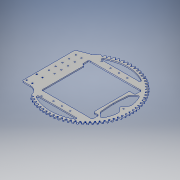
# Autodesk Inventor part: Bearing Plate
Saved by Autodesk Inventor 2019.4 (Build 234330000, 330)
## iProperties
Created: 2020-01-22
Part Number: Bearing Plate
Material: Aluminum 6061
Document SubType Name: Modeling
Designer: admin
Density: 2.7 g/cm^3
Appearance: Aluminum - Flat
Mass: 847.199 g
Surface Area: 1421.78 cm^2
Volume: 313.778 cm^3
Author: admin
Autodesk Inventor part; units mm, degrees
(part 1 of 6)
ref_plane "YZ Plane" through (0, 0, 0) normal (1, 0, 0) x (0, 1, 0)
ref_plane "XZ Plane" through (0, 0, 0) normal (0, 1, 0) x (-1, 0, 0)
ref_plane "XY Plane" through (0, 0, 0) normal (0, 0, 1) x (1, 0, 0)
sketch "Sketch1" plane through (0, 0, 0) normal (0, 1, 0) x (-1, 0, 0)
  arc A0 (63.1453, -163.2105) -> (129.2323, 118) centre (0, 0) ccw construction
  circle A1 centre (0, 0) radius 101.6 construction
  line L0 (-100.2, 110.3) -> (100.2, 110.3)
  line L1 (100.2, 110.3) -> (100.2, -110.3)
  line L2 (100.2, -110.3) -> (-100.2, -110.3)
  line L3 (-100.2, -110.3) -> (-100.2, 110.3)
  line L4 (-100.2, 110.3) -> (100.2, -110.3) construction
  line L5 (100.2, 110.3) -> (-100.2, -110.3) construction
  line L6 (180, 118) -> (180, -118)
  line L7 (180, -118) -> (63.1453, -163.2105)
  line L8 (180, 0) -> (0, 0)
  line L9 (180, 118) -> (129.2323, 118)
  arc A2 (129.2323, 118) -> (63.1453, -163.2105) centre (0, 0) ccw
  dimension "d0" = 350
  dimension "d1" = 203.2
  dimension "d4" = 220.6
  dimension "d5" = 200.4
  dimension "d6" = 180
  dimension "d7" = 118
  constraints: 20 end point, 4 point on circle, 3 centre point, 3 midpoint, 2 coincident, 2 horizontal, 2 parallel, 2 perpendicular, 1 tangent, 1 vertical
  measures "d0" diameter of A0
  measures "d1" diameter of A1
  measures "d4" distance of L2.end L0.start
  measures "d5" distance of L0.start L0.end
  measures "d6" distance from line of point (0, 0) L6
  measures "d7" distance from line of point (0, 0) L9
extrude "Extrusion1" add sketch "Sketch1" along normal blind 5
sketch "Sketch2" plane through (0, 0, 0) normal (0, -1, 0) x (1, 0, 0)
  circle A0 centre (-172.1762, 60.275) radius 2.0193 construction
  circle A1 centre (-172.1762, 105.1064) radius 2.0193 construction
  circle A2 centre (-146.7762, 105.1064) radius 2.0193 construction
  circle A3 centre (-146.7762, 60.275) radius 2.0193 construction
  circle A4 centre (-172.1762, 105.1064) radius 3
  circle A5 centre (-146.7762, 105.1064) radius 3
  circle A6 centre (-146.7762, 60.275) radius 3
  circle A7 centre (-172.1762, 60.275) radius 3
  point P0 (0, 0)
  dimension "d75" = 6
  dimension "d76" = 6
  dimension "d77" = 6
  dimension "d78" = 6
  constraints: 4 centre point, 4 coincident
  measures "d75" diameter of A4
  measures "d76" diameter of A5
  measures "d77" diameter of A6
  measures "d78" diameter of A7
extrude "Extrusion2" cut sketch "Sketch2" against normal through all
chamfer "Chamfer1" distance 3 angle 45 4 edges at (-175.1762, 0, 60.275) (-149.7762, 0, 60.275) (-149.7762, 0, 105.1064) (-175.1762, 0, 105.1064)
sketch "Sketch3" plane through (0, 5, 0) normal (0, 1, 0) x (1, 0, 0)
  line L0 (154.7299, 0) -> (-77.3649, -134) construction
  line L1 (-77.3649, -134) -> (-77.3649, 134) construction
  line L2 (-77.3649, 134) -> (154.7299, 0) construction
  circle A0 centre (-77.3649, 134) radius 2.75
  circle A1 centre (-77.3649, -134) radius 2.75
  circle A2 centre (154.7299, 0) radius 2.75
  point P0 (0, 0)
  point P1 (0, 0)
  dimension "d17" = 268
  dimension "d18" = 5.5
  dimension "d19" = 5.5
  dimension "d20" = 5.5
  constraints: 6 end point, 4 coincident, 3 centre point, 1 vertical, 7 other
  measures "d17" distance of L1.end L0.start
  measures "d18" diameter of A0
  measures "d19" diameter of A1
  measures "d20" diameter of A2
extrude "Extrusion3" cut sketch "Sketch3" against normal through all
sketch "Sketch4" plane through (0, 5, 0) normal (0, 1, 0) x (1, 0, 0)
  circle A0 centre (0, 0) radius 191.0078 construction
  arc A1 (190.8769, -4.9983) -> (190.3537, -14.9812) centre (190.746, -9.9966) ccw
  arc A2 (190.746, -9.9966) -> (201.0078, 0) centre (191.0078, 0) ccw
  arc A3 (199.9066, -21.011) -> (190.746, -9.9966) centre (189.9614, -19.9657) ccw
  line L0 (0, 0) -> (199.9066, -21.011) construction
  arc A4 (189.3088, -24.923) -> (193.6558, -29.9343) centre (188.6561, -29.8802) ccw construction
  line L1 (0, 0) -> (201.0078, 0)
  arc A5 (195.7441, 9.8581) -> (190.8769, 4.9983) centre (190.746, 9.9966) ccw construction
  arc A6 (189.3088, -24.923) -> (190.3537, -14.9812) centre (189.9614, -19.9657) ccw
  arc A7 (190.8769, -4.9983) -> (190.8769, 4.9983) centre (191.0078, 0) ccw
  arc A8 (-129.2323, -118) -> (-63.1453, 163.2105) centre (0, 0) ccw projected
  line L2 (196.0078, 0) -> (175, 0)
  line L3 (194.934, -20.4884) -> (174.0413, -18.2925)
  arc A9 (201.0078, 0) -> (190.746, 9.9966) centre (191.0078, 0) ccw
  arc A10 (190.746, 9.9966) -> (199.9066, 21.011) centre (189.9614, 19.9657) ccw
  arc A11 (199.9066, 21.011) -> (188.6561, 29.8802) centre (189.9614, 19.9657) ccw
  arc A12 (188.6561, 29.8802) -> (196.6152, 41.7919) centre (186.8338, 39.7127) ccw
  arc A13 (196.6152, 41.7919) -> (184.4993, 49.4364) centre (186.8338, 39.7127) ccw
  arc A14 (184.4993, 49.4364) -> (191.1697, 62.1148) centre (181.6592, 59.0246) ccw
  arc A15 (191.1697, 62.1148) -> (178.3211, 68.4511) centre (181.6592, 59.0246) ccw
  arc A16 (178.3211, 68.4511) -> (183.6297, 81.7572) centre (174.4943, 77.6899) ccw
  arc A17 (183.6297, 81.7572) -> (170.1892, 86.7157) centre (174.4943, 77.6899) ccw
  arc A18 (170.1892, 86.7157) -> (174.0778, 100.5039) centre (165.4176, 95.5039) ccw
  arc A19 (174.0778, 100.5039) -> (160.1926, 104.0303) centre (165.4176, 95.5039) ccw
  arc A20 (160.1926, 104.0303) -> (162.6187, 118.1494) centre (154.5285, 112.2715) ccw
  arc A21 (162.6187, 118.1494) -> (148.4409, 120.2051) centre (154.5285, 112.2715) ccw
  arc A22 (148.4409, 120.2051) -> (149.3779, 134.5004) centre (141.9464, 127.8091) ccw
  arc A23 (149.3779, 134.5004) -> (135.0629, 135.0629) centre (141.9464, 127.8091) ccw
  arc A24 (135.0629, 135.0629) -> (134.5004, 149.3779) centre (127.8091, 141.9464) ccw
  arc A25 (134.5004, 149.3779) -> (120.2051, 148.4409) centre (127.8091, 141.9464) ccw
  arc A26 (120.2051, 148.4409) -> (118.1494, 162.6187) centre (112.2715, 154.5285) ccw
  arc A27 (118.1494, 162.6187) -> (104.0303, 160.1926) centre (112.2715, 154.5285) ccw
  arc A28 (104.0303, 160.1926) -> (100.5039, 174.0778) centre (95.5039, 165.4176) ccw
  arc A29 (100.5039, 174.0778) -> (86.7157, 170.1892) centre (95.5039, 165.4176) ccw
  arc A30 (86.7157, 170.1892) -> (81.7572, 183.6297) centre (77.6899, 174.4943) ccw
  arc A31 (81.7572, 183.6297) -> (68.4511, 178.3211) centre (77.6899, 174.4943) ccw
  arc A32 (68.4511, 178.3211) -> (62.1148, 191.1697) centre (59.0246, 181.6592) ccw
  arc A33 (62.1148, 191.1697) -> (49.4364, 184.4993) centre (59.0246, 181.6592) ccw
  arc A34 (49.4364, 184.4993) -> (41.7919, 196.6152) centre (39.7127, 186.8338) ccw
  arc A35 (41.7919, 196.6152) -> (29.8802, 188.6561) centre (39.7127, 186.8338) ccw
  arc A36 (29.8802, 188.6561) -> (21.011, 199.9066) centre (19.9657, 189.9614) ccw
  arc A37 (21.011, 199.9066) -> (9.9966, 190.746) centre (19.9657, 189.9614) ccw
  arc A38 (9.9966, 190.746) -> (0, 201.0078) centre (0, 191.0078) ccw
  arc A39 (0, 201.0078) -> (-9.9966, 190.746) centre (0, 191.0078) ccw
  arc A40 (-9.9966, 190.746) -> (-21.011, 199.9066) centre (-19.9657, 189.9614) ccw
  arc A41 (-21.011, 199.9066) -> (-29.8802, 188.6561) centre (-19.9657, 189.9614) ccw
  arc A42 (-29.8802, 188.6561) -> (-41.7919, 196.6152) centre (-39.7127, 186.8338) ccw
  arc A43 (-41.7919, 196.6152) -> (-49.4364, 184.4993) centre (-39.7127, 186.8338) ccw
  arc A44 (-49.4364, 184.4993) -> (-62.1148, 191.1697) centre (-59.0246, 181.6592) ccw
  arc A45 (-62.1148, 191.1697) -> (-68.4511, 178.3211) centre (-59.0246, 181.6592) ccw
  arc A46 (-68.4511, 178.3211) -> (-81.7572, 183.6297) centre (-77.6899, 174.4943) ccw
  arc A47 (-81.7572, 183.6297) -> (-86.7157, 170.1892) centre (-77.6899, 174.4943) ccw
  arc A48 (-86.7157, 170.1892) -> (-100.5039, 174.0778) centre (-95.5039, 165.4176) ccw
  arc A49 (196.3819, -42.8749) -> (188.4886, -30.9195) centre (186.6121, -40.7419) ccw
  arc A50 (188.4886, -30.9195) -> (199.7878, -22.1125) centre (189.8485, -21.0124) ccw
  arc A51 (190.4734, -64.2183) -> (183.9432, -51.4672) centre (180.9975, -61.0235) ccw
  arc A52 (183.9432, -51.4672) -> (196.1426, -43.9566) centre (186.3847, -41.7698) ccw
  arc A53 (182.2528, -84.7822) -> (177.165, -71.39) centre (173.1859, -80.5643) ccw
  arc A54 (177.165, -71.39) -> (190.1166, -65.2671) centre (180.6584, -62.0201) ccw
  arc A55 (171.82, -104.3169) -> (168.2362, -90.4464) centre (163.272, -99.1272) ccw
  arc A56 (168.2362, -90.4464) -> (181.7828, -85.7854) centre (172.7392, -81.5176) ccw
  arc A57 (159.3014, -122.5854) -> (157.2653, -108.4048) centre (151.3763, -116.4868) ccw
  arc A58 (157.2653, -108.4048) -> (171.2424, -105.2623) centre (162.7232, -100.0256) ccw
  arc A59 (144.8492, -139.3658) -> (144.3854, -125.0473) centre (137.643, -132.4325) ccw
  arc A60 (144.3854, -125.0473) -> (158.6234, -123.4615) centre (150.732, -117.3194) ccw
  arc A61 (128.6386, -154.4546) -> (129.7528, -140.1719) centre (122.239, -146.7706) ccw
  arc A62 (129.7528, -140.1719) -> (144.0788, -140.1621) centre (136.911, -133.1891) ccw
  arc A63 (110.8666, -167.6685) -> (113.5452, -153.5951) centre (105.3511, -159.3271) ccw
  arc A64 (113.5452, -153.5951) -> (127.7854, -155.1612) centre (121.4282, -147.4421) ccw
  arc A65 (91.7488, -178.8471) -> (95.9594, -165.1537) centre (87.1844, -169.9495) ccw
  arc A66 (95.9594, -165.1537) -> (109.9408, -168.277) centre (104.4713, -159.9053) ccw
  arc A67 (71.5173, -187.8547) -> (77.2087, -174.7077) centre (67.9594, -178.5091) ccw
  arc A68 (77.2087, -174.7077) -> (90.7617, -179.35) centre (86.2464, -170.4275) ccw
  arc A69 (50.4177, -194.582) -> (57.5208, -182.1409) centre (47.9095, -184.9017) ccw
  arc A70 (57.5208, -182.1409) -> (70.4809, -188.246) centre (66.9745, -178.8809) ccw
  arc A71 (28.7061, -198.9474) -> (37.1347, -187.3632) centre (27.278, -189.0499) ccw
  arc A72 (37.1347, -187.3632) -> (49.3445, -194.857) centre (46.8896, -185.163) ccw
  arc A73 (6.646, -200.8979) -> (16.2978, -190.3112) centre (6.3154, -190.9033) ccw
  arc A74 (16.2978, -190.3112) -> (27.6091, -199.1026) centre (26.2356, -189.1974) ccw
  arc A75 (-15.4948, -200.4097) -> (-4.7369, -190.949) centre (-14.7239, -190.4394) ccw
  arc A76 (-4.7369, -190.949) -> (5.5386, -200.9314) centre (5.2631, -190.9352) ccw
  arc A77 (-37.4474, -197.4887) -> (-25.7141, -189.269) centre (-35.5844, -187.6638) ccw
  arc A78 (-25.7141, -189.269) -> (-16.5991, -200.3212) centre (-15.7733, -190.3554) ccw
  arc A79 (-58.9455, -192.1706) -> (-46.3792, -185.2915) centre (-56.013, -182.6102) ccw
  arc A80 (-46.3792, -185.2915) -> (-38.5353, -197.2794) centre (-36.6182, -187.4648) ccw
  arc A81 (-79.7281, -184.5198) -> (-66.4813, -179.0648) centre (-75.7617, -175.34) ccw
  arc A82 (-66.4813, -179.0648) -> (-60.0038, -191.8428) centre (-57.0186, -182.2988) ccw
  arc A83 (-99.5429, -174.6291) -> (-85.7764, -170.6645) centre (-94.5907, -165.9414) ccw
  arc A84 (-85.7764, -170.6645) -> (-80.7439, -184.0775) centre (-76.7269, -174.9198) ccw
  arc A85 (-118.1494, -162.6187) -> (-104.0303, -160.1926) centre (-112.2715, -154.5285) ccw
  arc A86 (-104.0303, -160.1926) -> (-100.5039, -174.0778) centre (-95.5039, -165.4176) ccw
  circle A87 centre (154.7299, 0) radius 2.75 projected
  line L4 (154.7299, 0) -> (-77.3649, -134) construction
  line L5 (-77.3649, -134) -> (-77.3649, 134) construction
  line L6 (-77.3649, 134) -> (154.7299, 0) construction
  circle A88 centre (-77.3649, 134) radius 2.75 projected
  circle A89 centre (-77.3649, -134) radius 2.75 projected
  point P0 (0, 0)
  dimension "d24" = 5
  dimension "d28" = 5
  dimension "d30" = 6
  dimension "d31" = 5
  dimension "d32" = 5
  dimension "d33" = 5
  dimension "d45" = 120
  dimension "d49" = 120
  constraints: 179 point on circle, 86 centre point, 14 end point, 4 coincident, 4 equal radius, 4 point on line, 1 horizontal, 282 other
  measures "d24" radius of A1
  measures "d28" radius of A4
  measures "d30" angle of L0 L1
  measures "d31" radius of A5
  measures "d32" radius of A6
  measures "d33" radius of A7
extrude "Extrusion4" [suppressed]
pattern_circular "Circular Pattern1" [suppressed]
sketch "Sketch5" plane through (0, 5, 0) normal (0, 1, 0) x (1, 0, 0)
  line L0 (-115.2105, -158.5736) -> (-122.0328, -125.4312)
  arc A0 (-91.1098, 167.8034) -> (-98.0039, 169.7477) centre (-95.5039, 165.4176) ccw projected
  line L1 (-98.0039, 169.7477) -> (-112.1506, 144.2506)
  line L2 (-63.1453, 163.2105) -> (-180, 118) projected
  line L3 (-88.554, 153.38) -> (-98.0039, 169.7477)
  arc A1 (-129.2323, -118) -> (-63.1453, 163.2105) centre (0, 0) ccw projected
  line L4 (-115.2105, -158.5736) -> (-102.8624, -141.578) projected
  dimension "d51" = 25
  dimension "d52" = 25
  constraints: 6 end point, 1 point on circle, 1 point on line
  measures "d51" distance from line of L4 L0.end
  measures "d52" distance from line of L3 L1.end
extrude "Extrusion5" [suppressed]
sketch "Sketch6" plane through (0, 5, 0) normal (0, 1, 0) x (1, 0, 0)
  line L0 (-100.2, -110.3) -> (-100.2, 110.3) projected
  line L1 (-100.2, 110.3) -> (-110.2, 110.3)
  line L2 (-110.2, 110.3) -> (-110.2, 80.3)
  line L3 (-110.2, 80.3) -> (-100.2, 80.3)
  point P0 (0, 0)
  dimension "d59" = 30
  dimension "d60" = 10
  constraints: 6 end point, 2 perpendicular, 1 horizontal, 1 point on line
  measures "d59" distance of L1.end L2.end
  measures "d60" distance of L2.end L3.end
extrude "Extrusion6" cut sketch "Sketch6" against normal through all
sketch "Sketch10" plane through (0, 5, 0) normal (0, 1, 0) x (1, 0, 0)
  line L0 (100.2, -110.3) -> (125.2, -110.3)
  line L1 (125.2, -110.3) -> (125.2, -80.3)
  line L2 (125.2, -80.3) -> (100.2, -80.3)
  line L3 (100.2, -110.3) -> (100.2, 110.3) projected
  point P0 (0, 0)
  dimension "d81" = 30
  dimension "d82" = 25
  constraints: 6 end point, 2 perpendicular, 1 horizontal, 1 point on line
  measures "d81" distance of L0.end L1.end
  measures "d82" distance of L0.start L0.end
extrude "Extrusion8" cut sketch "Sketch10" against normal through all
mirror "Mirror1" about plane through (0, 0, 0) normal (0, 0, 1) of "Extrusion8"
fillet "Fillet1" radius 5 9 edges at (-110.2, 2.5, -110.3) (-110.2, 2.5, -80.3) (-100.2, 2.5, -80.3) (100.2, 2.5, 80.3) (125.2, 2.5, 80.3) (125.2, 2.5, 110.3) (100.2, 2.5, -80.3) (125.2, 2.5, -80.3) (125.2, 2.5, -110.3)
fillet "Fillet2" [suppressed]
fillet "Fillet3" radius 2.5 1 edges at (-100.2, 2.5, 110.3)
fillet "Fillet4" radius 5 2 edges at (-180, 2.5, 118) (-180, 2.5, -118)
sketch "Sketch8" plane through (0, 5, 0) normal (0, 1, 0) x (1, 0, 0)
  arc A0 (-100.2, 75.3) -> (-105.2, 80.3) centre (-105.2, 75.3) ccw projected
  arc A1 (-110.2, 85.3) -> (-105.2, 80.3) centre (-105.2, 85.3) ccw projected
  line L0 (-110.2, 85.3) -> (-110.2, 105.3) projected
  arc A2 (-105.2, 110.3) -> (-110.2, 105.3) centre (-105.2, 105.3) ccw projected
  line L1 (-105.2, 110.3) -> (120.2, 110.3) projected
  line L2 (100.2, 75.3) -> (100.2, -75.3) projected
  line L3 (120.2, -110.3) -> (-97.7, -110.3) projected
  arc A3 (-100.2, -107.8) -> (-97.7, -110.3) centre (-97.7, -107.8) ccw projected
  line L4 (-100.2, -107.8) -> (-100.2, 75.3) projected
  circle A4 centre (154.7299, 0) radius 2.75 projected
  circle A5 centre (-77.3649, 134) radius 2.75 projected
  circle A6 centre (-77.3649, -134) radius 2.75 projected
  arc A7 (-176.8042, 119.2365) -> (-180, 114.5733) centre (-175, 114.5733) ccw projected
  line L5 (-180, 114.5733) -> (-180, -113) projected
  arc A8 (-180, -113) -> (-175, -118) centre (-175, -113) ccw projected
  line L6 (-175, -118) -> (-129.2323, -118) projected
  arc A9 (-129.2323, -118) -> (-63.1453, 163.2105) centre (0, 0) ccw projected
  line L7 (-63.1453, 163.2105) -> (-176.8042, 119.2365) projected
  line L8 (-185, -113) -> (-185, 114.5733)
  arc A10 (-178.6083, 123.8996) -> (-185, 114.5733) centre (-175, 114.5733) ccw
  line L9 (-178.6083, 123.8996) -> (-115.644, 148.2602)
  line L10 (-115.644, 148.2602) -> (-102.6825, 171.6211)
  arc A11 (-99.0294, 174.7755) -> (-102.6825, 171.6211) centre (-96.5615, 168.2249) ccw
  arc A12 (-86.7157, 170.1892) -> (-99.0294, 174.7755) centre (-95.5039, 165.4176) ccw
  arc A13 (-68.4511, 178.3211) -> (-86.7157, 170.1892) centre (-77.6899, 174.4943) ccw
  arc A14 (-49.4364, 184.4993) -> (-68.4511, 178.3211) centre (-59.0246, 181.6592) ccw
  arc A15 (-29.8802, 188.6561) -> (-49.4364, 184.4993) centre (-39.7127, 186.8338) ccw
  arc A16 (-9.9966, 190.746) -> (-29.8802, 188.6561) centre (-19.9657, 189.9614) ccw
  arc A17 (9.9966, 190.746) -> (-9.9966, 190.746) centre (0, 191.0078) ccw
  arc A18 (29.8802, 188.6561) -> (9.9966, 190.746) centre (19.9657, 189.9614) ccw
  arc A19 (49.4364, 184.4993) -> (29.8802, 188.6561) centre (39.7127, 186.8338) ccw
  arc A20 (68.4511, 178.3211) -> (49.4364, 184.4993) centre (59.0246, 181.6592) ccw
  arc A21 (86.7157, 170.1892) -> (68.4511, 178.3211) centre (77.6899, 174.4943) ccw
  arc A22 (104.0303, 160.1926) -> (86.7157, 170.1892) centre (95.5039, 165.4176) ccw
  arc A23 (120.2051, 148.4409) -> (104.0303, 160.1926) centre (112.2715, 154.5285) ccw
  arc A24 (135.0629, 135.0629) -> (120.2051, 148.4409) centre (127.8091, 141.9464) ccw
  arc A25 (148.4409, 120.2051) -> (135.0629, 135.0629) centre (141.9464, 127.8091) ccw
  arc A26 (160.1926, 104.0303) -> (148.4409, 120.2051) centre (154.5285, 112.2715) ccw
  arc A27 (170.1892, 86.7157) -> (160.1926, 104.0303) centre (165.4176, 95.5039) ccw
  arc A28 (178.3211, 68.4511) -> (170.1892, 86.7157) centre (174.4943, 77.6899) ccw
  arc A29 (184.4993, 49.4364) -> (178.3211, 68.4511) centre (181.6592, 59.0246) ccw
  arc A30 (188.6561, 29.8802) -> (184.4993, 49.4364) centre (186.8338, 39.7127) ccw
  arc A31 (190.746, 9.9966) -> (188.6561, 29.8802) centre (189.9614, 19.9657) ccw
  arc A32 (190.746, -9.9966) -> (190.746, 9.9966) centre (191.0078, 0) ccw
  arc A33 (188.6561, -29.8802) -> (190.746, -9.9966) centre (189.9614, -19.9657) ccw
  arc A34 (184.4993, -49.4364) -> (188.6561, -29.8802) centre (186.8338, -39.7127) ccw
  arc A35 (178.3211, -68.4511) -> (184.4993, -49.4364) centre (181.6592, -59.0246) ccw
  arc A36 (170.1892, -86.7157) -> (178.3211, -68.4511) centre (174.4943, -77.6899) ccw
  arc A37 (160.1926, -104.0303) -> (170.1892, -86.7157) centre (165.4176, -95.5039) ccw
  arc A38 (148.4409, -120.2051) -> (160.1926, -104.0303) centre (154.5285, -112.2715) ccw
  arc A39 (135.0629, -135.0629) -> (148.4409, -120.2051) centre (141.9464, -127.8091) ccw
  arc A40 (120.2051, -148.4409) -> (135.0629, -135.0629) centre (127.8091, -141.9464) ccw
  arc A41 (104.0303, -160.1926) -> (120.2051, -148.4409) centre (112.2715, -154.5285) ccw
  arc A42 (86.7157, -170.1892) -> (104.0303, -160.1926) centre (95.5039, -165.4176) ccw
  arc A43 (68.4511, -178.3211) -> (86.7157, -170.1892) centre (77.6899, -174.4943) ccw
  arc A44 (49.4364, -184.4993) -> (68.4511, -178.3211) centre (59.0246, -181.6592) ccw
  arc A45 (29.8802, -188.6561) -> (49.4364, -184.4993) centre (39.7127, -186.8338) ccw
  arc A46 (9.9966, -190.746) -> (29.8802, -188.6561) centre (19.9657, -189.9614) ccw
  arc A47 (-9.9966, -190.746) -> (9.9966, -190.746) centre (0, -191.0078) ccw
  arc A48 (-29.8802, -188.6561) -> (-9.9966, -190.746) centre (-19.9657, -189.9614) ccw
  arc A49 (-49.4364, -184.4993) -> (-29.8802, -188.6561) centre (-39.7127, -186.8338) ccw
  arc A50 (-68.4511, -178.3211) -> (-49.4364, -184.4993) centre (-59.0246, -181.6592) ccw
  arc A51 (-86.7157, -170.1892) -> (-68.4511, -178.3211) centre (-77.6899, -174.4943) ccw
  arc A52 (-104.0303, -160.1926) -> (-86.7157, -170.1892) centre (-95.5039, -165.4176) ccw
  arc A53 (-116.1388, -163.7505) -> (-104.0303, -160.1926) centre (-112.2715, -154.5285) ccw
  arc A54 (-120.288, -158.7065) -> (-116.1388, -163.7505) centre (-113.4317, -157.2951) ccw
  line L11 (-120.288, -158.7065) -> (-126.6228, -127.9323)
  arc A55 (-131.4192, -123) -> (-126.6228, -127.9323) centre (0, 0) ccw
  line L12 (-131.4192, -123) -> (-175, -123)
  arc A56 (-185, -113) -> (-175, -123) centre (-175, -113) ccw
  arc A57 (-95.2, 75.3) -> (-105.2, 85.3) centre (-105.2, 75.3) ccw
  line L13 (-105.2, 85.3) -> (-105.2, 105.3)
  line L14 (-105.2, 105.3) -> (95.2, 105.3)
  line L15 (95.2, 105.3) -> (95.2, -105.3)
  line L16 (95.2, -105.3) -> (-95.2, -105.3)
  line L17 (-95.2, -105.3) -> (-95.2, 75.3)
  arc A58 (100.2, -75.3) -> (105.2, -80.3) centre (105.2, -75.3) ccw projected
  line L18 (105.2, -80.3) -> (120.2, -80.3) projected
  arc A59 (125.2, -85.3) -> (120.2, -80.3) centre (120.2, -85.3) ccw projected
  line L19 (125.2, -85.3) -> (125.2, -105.3) projected
  arc A60 (120.2, -110.3) -> (125.2, -105.3) centre (120.2, -105.3) ccw projected
  line L20 (125.2, 105.3) -> (125.2, 85.3) projected
  line L21 (120.2, 80.3) -> (105.2, 80.3) projected
  arc A61 (105.2, 80.3) -> (100.2, 75.3) centre (105.2, 75.3) ccw projected
  arc A62 (125.2, 105.3) -> (120.2, 110.3) centre (120.2, 105.3) ccw projected
  arc A63 (120.2, 80.3) -> (125.2, 85.3) centre (120.2, 85.3) ccw projected
  dimension "d69" = 5
  dimension "d70" = 5
  constraints: 96 point on circle, 48 centre point, 20 end point, 9 other
  measures "d69" distance between parallel lines of L5 L8
  measures "d70" distance between parallel lines of L4 L17
sketch "Sketch9" plane through (0, 5, 0) normal (0, 1, 0) x (1, 0, 0)
  circle A0 centre (-30.7, -127.3) radius 2.75 projected
  circle A1 centre (6.8, -127.3) radius 2.75 projected
  circle A2 centre (44.3, -127.3) radius 2.75 projected
  circle A3 centre (-30.7, 127.3) radius 2.75 projected
  circle A4 centre (6.8, 127.3) radius 2.75 projected
  circle A5 centre (44.3, 127.3) radius 2.75 projected
  point P0 (0, 0)
extrude "Extrusion7" cut sketch "Sketch9" against normal through all
sketch "Sketch11" plane through (0, 5, 0) normal (0, 1, 0) x (1, 0, 0)
  circle A0 centre (-135, 102) radius 2.75
  circle A1 centre (-160, 102) radius 2.75
  line L0 (-175, -118) -> (-129.2323, -118) projected
  line L1 (-180, 114.5733) -> (-180, -113) projected
  circle A2 centre (-160, 72) radius 2.75
  circle A3 centre (-135, 72) radius 2.75
  circle A4 centre (-160, 42) radius 2.75
  circle A5 centre (-135, 42) radius 2.75
  circle A6 centre (-160, 12) radius 2.75
  circle A7 centre (-135, 12) radius 2.75
  circle A8 centre (-160, -18) radius 2.75
  circle A9 centre (-135, -18) radius 2.75
  point P0 (0, 0)
  dimension "d85" = 5.5
  dimension "d86" = 5.5
  dimension "d87" = 25
  dimension "d88" = 220
  dimension "d89" = 220
  dimension "d90" = 20
  dimension "d93" = 30
  constraints: 10 centre point, 1 vertical, 16 other
  measures "d85" diameter of A0
  measures "d86" diameter of A1
  measures "d87" distance of A0.centre A1.centre
  measures "d88" distance from line of L0 A1.centre
  measures "d89" distance from line of L0 A0.centre
  measures "d90" distance from line of L1 A1.centre
  measures "d93" distance of A1.centre A2.centre
extrude "Extrusion9" cut sketch "Sketch11" against normal blind 10
sketch "Sketch12" plane through (0, 5, 0) normal (0, 1, 0) x (1, 0, 0)
  arc A0 (21.9852, -177.5935) -> (23.4739, -177.4029) centre (0, 0) ccw
  spline S0 degree 3 poles (25.1414, -178.3516) (25.0255, -178.0811) (24.5751, -177.5264) (23.8629, -177.3514) (23.4739, -177.4029) knots 0 0 0 0 0.428571 1 1 1 1
  spline S1 degree 5 poles (25.1414, -178.3516) (25.1443, -178.3585) (25.1662, -178.4095) (25.2071, -178.5046) (25.2675, -178.6437) (25.3477, -178.8267) (25.4454, -179.0467) (25.5442, -179.2663) (25.6441, -179.4856) (25.7451, -179.7045) (25.8472, -179.9232) (25.9503, -180.1416) (26.0546, -180.3596) (26.1598, -180.5773) (26.2661, -180.7947) (26.3734, -181.0119) (26.4817, -181.2287) (26.5909, -181.4452) (26.7012, -181.6614) (26.8124, -181.8773) (26.9246, -182.0928) (27.0377, -182.3081) (27.1517, -182.5231) (27.2667, -182.7378) (27.3826, -182.9522) (27.4994, -183.1663) (27.617, -183.38) (27.7356, -183.5935) (27.8551, -183.8067) (27.9754, -184.0196) (28.0966, -184.2322) (28.2187, -184.4444) (28.3416, -184.6564) (28.4653, -184.8681) (28.5899, -185.0795) (28.7153, -185.2906) (28.8415, -185.5014) (28.9686, -185.7119) (29.0964, -185.9221) (29.2251, -186.132) (29.3545, -186.3416) (29.4848, -186.5509) (29.6158, -186.7599) (29.774, -187.0104) (29.9068, -187.2187) (30.0136, -187.3852) (30.0941, -187.5098) (30.1479, -187.5929) knots 0.383497 0.383497 0.383497 0.383497 0.383497 0.383497 0.385714 0.4 0.414286 0.428571 0.442857 0.457143 0.471429 0.485714 0.5 0.514286 0.528571 0.542857 0.557143 0.571429 0.585714 0.6 0.614286 0.628571 0.642857 0.657143 0.671429 0.685714 0.7 0.714286 0.728571 0.742857 0.757143 0.771429 0.785714 0.8 0.814286 0.828571 0.842857 0.857143 0.871429 0.885714 0.9 0.914286 0.928571 0.942857 0.957143 0.971429 1 1 1 1 1 1
  arc A1 (30.1479, -187.5929) -> (34.0689, -186.9206) centre (0, 0) ccw
  spline S2 degree 5 poles (35.7108, -176.5393) (35.7103, -176.5467) (35.7067, -176.6021) (35.6998, -176.7054) (35.6892, -176.8567) (35.6746, -177.056) (35.6557, -177.2959) (35.6357, -177.5359) (35.6146, -177.776) (35.5923, -178.0161) (35.5688, -178.2563) (35.5443, -178.4965) (35.5187, -178.7368) (35.492, -178.9772) (35.4642, -179.2176) (35.4354, -179.458) (35.4055, -179.6985) (35.3746, -179.9391) (35.3427, -180.1796) (35.3097, -180.4202) (35.2758, -180.6609) (35.2409, -180.9015) (35.205, -181.1422) (35.1681, -181.383) (35.1302, -181.6237) (35.0914, -181.8645) (35.0517, -182.1052) (35.011, -182.346) (34.9694, -182.5868) (34.9269, -182.8276) (34.8834, -183.0684) (34.8391, -183.3093) (34.7938, -183.5501) (34.7476, -183.7909) (34.7006, -184.0317) (34.6527, -184.2725) (34.6039, -184.5133) (34.5542, -184.7541) (34.5037, -184.9949) (34.4523, -185.2357) (34.4001, -185.4764) (34.347, -185.7172) (34.2931, -185.9579) (34.2274, -186.2468) (34.1716, -186.4874) (34.1263, -186.68) (34.092, -186.8243) (34.0689, -186.9206) knots 0.383497 0.383497 0.383497 0.383497 0.383497 0.383497 0.385714 0.4 0.414286 0.428571 0.442857 0.457143 0.471429 0.485714 0.5 0.514286 0.528571 0.542857 0.557143 0.571429 0.585714 0.6 0.614286 0.628571 0.642857 0.657143 0.671429 0.685714 0.7 0.714286 0.728571 0.742857 0.757143 0.771429 0.785714 0.8 0.814286 0.828571 0.842857 0.857143 0.871429 0.885714 0.9 0.914286 0.928571 0.942857 0.957143 0.971429 1 1 1 1 1 1
  spline S3 degree 3 poles (36.967, -175.0893) (36.583, -175.1703) (35.9698, -175.5726) (35.7299, -176.2456) (35.7108, -176.5393) knots 0 0 0 0 0.571429 1 1 1 1
  arc A2 (36.967, -175.0893) -> (38.4341, -174.7731) centre (0, 0) ccw
  spline S4 degree 3 poles (40.1761, -175.577) (40.0377, -175.3172) (39.5419, -174.8028) (38.8174, -174.6888) (38.4341, -174.7731) knots 0 0 0 0 0.428571 1 1 1 1
  spline S5 degree 5 poles (40.1761, -175.577) (40.1796, -175.5835) (40.2057, -175.6325) (40.2546, -175.7238) (40.3265, -175.8573) (40.4219, -176.0329) (40.5379, -176.2437) (40.655, -176.4542) (40.7731, -176.6642) (40.8924, -176.8738) (41.0126, -177.083) (41.1339, -177.2918) (41.2563, -177.5003) (41.3796, -177.7083) (41.5039, -177.9159) (41.6292, -178.1231) (41.7555, -178.33) (41.8828, -178.5364) (42.011, -178.7425) (42.1401, -178.9482) (42.2701, -179.1535) (42.4011, -179.3584) (42.5329, -179.5629) (42.6657, -179.7671) (42.7994, -179.9709) (42.9339, -180.1743) (43.0693, -180.3773) (43.2055, -180.58) (43.3426, -180.7823) (43.4806, -180.9842) (43.6194, -181.1857) (43.759, -181.3869) (43.8994, -181.5877) (44.0407, -181.7881) (44.1827, -181.9882) (44.3256, -182.1879) (44.4692, -182.3872) (44.6137, -182.5861) (44.7589, -182.7847) (44.9049, -182.983) (45.0517, -183.1809) (45.1992, -183.3784) (45.3475, -183.5755) (45.5263, -183.8117) (45.6763, -184.008) (45.7969, -184.1648) (45.8876, -184.2822) (45.9483, -184.3604) knots 0.383497 0.383497 0.383497 0.383497 0.383497 0.383497 0.385714 0.4 0.414286 0.428571 0.442857 0.457143 0.471429 0.485714 0.5 0.514286 0.528571 0.542857 0.557143 0.571429 0.585714 0.6 0.614286 0.628571 0.642857 0.657143 0.671429 0.685714 0.7 0.714286 0.728571 0.742857 0.757143 0.771429 0.785714 0.8 0.814286 0.828571 0.842857 0.857143 0.871429 0.885714 0.9 0.914286 0.928571 0.942857 0.957143 0.971429 1 1 1 1 1 1
  arc A3 (45.9483, -184.3604) -> (49.7981, -183.358) centre (0, 0) ccw
  spline S6 degree 5 poles (50.5537, -172.8748) (50.5538, -172.8823) (50.5549, -172.9378) (50.5568, -173.0413) (50.5591, -173.1929) (50.5614, -173.3928) (50.563, -173.6334) (50.5634, -173.8742) (50.5627, -174.1152) (50.5609, -174.3563) (50.5579, -174.5976) (50.5538, -174.8391) (50.5487, -175.0807) (50.5425, -175.3225) (50.5352, -175.5644) (50.5268, -175.8064) (50.5175, -176.0486) (50.5071, -176.2908) (50.4957, -176.5333) (50.4832, -176.7758) (50.4698, -177.0184) (50.4554, -177.2612) (50.4401, -177.5041) (50.4237, -177.7471) (50.4064, -177.9901) (50.3882, -178.2333) (50.369, -178.4766) (50.3489, -178.72) (50.3279, -178.9634) (50.3059, -179.207) (50.283, -179.4506) (50.2593, -179.6943) (50.2346, -179.9381) (50.209, -180.182) (50.1826, -180.4259) (50.1552, -180.6699) (50.127, -180.914) (50.098, -181.1581) (50.0681, -181.4024) (50.0373, -181.6466) (50.0056, -181.8909) (49.9732, -182.1353) (49.9399, -182.3797) (49.8989, -182.6731) (49.8637, -182.9177) (49.8349, -183.1133) (49.813, -183.2601) (49.7981, -183.358) knots 0.383497 0.383497 0.383497 0.383497 0.383497 0.383497 0.385714 0.4 0.414286 0.428571 0.442857 0.457143 0.471429 0.485714 0.5 0.514286 0.528571 0.542857 0.557143 0.571429 0.585714 0.6 0.614286 0.628571 0.642857 0.657143 0.671429 0.685714 0.7 0.714286 0.728571 0.742857 0.757143 0.771429 0.785714 0.8 0.814286 0.828571 0.842857 0.857143 0.871429 0.885714 0.9 0.914286 0.928571 0.942857 0.957143 0.971429 1 1 1 1 1 1
  spline S7 degree 3 poles (51.6824, -171.3235) (51.3067, -171.4368) (50.7298, -171.8896) (50.5479, -172.5806) (50.5537, -172.8748) knots 0 0 0 0 0.571429 1 1 1 1
  arc A4 (51.6824, -171.3235) -> (53.1175, -170.884) centre (0, 0) ccw
  spline S8 degree 3 poles (54.9213, -171.5373) (54.7614, -171.2902) (54.2237, -170.8197) (53.4922, -170.7676) (53.1175, -170.884) knots 0 0 0 0 0.428571 1 1 1 1
  spline S9 degree 5 poles (54.9213, -171.5373) (54.9254, -171.5435) (54.9555, -171.5901) (55.012, -171.6769) (55.0949, -171.8039) (55.2049, -171.9707) (55.3384, -172.171) (55.4729, -172.3707) (55.6084, -172.57) (55.745, -172.7687) (55.8826, -172.967) (56.0211, -173.1648) (56.1607, -173.362) (56.3012, -173.5589) (56.4427, -173.7552) (56.5852, -173.951) (56.7285, -174.1464) (56.8728, -174.3414) (57.018, -174.5358) (57.1641, -174.7298) (57.3111, -174.9233) (57.459, -175.1164) (57.6077, -175.309) (57.7573, -175.5012) (57.9078, -175.6929) (58.0591, -175.8842) (58.2112, -176.075) (58.3641, -176.2653) (58.5179, -176.4553) (58.6725, -176.6448) (58.8278, -176.8338) (58.984, -177.0224) (59.141, -177.2106) (59.2987, -177.3983) (59.4572, -177.5856) (59.6165, -177.7724) (59.7765, -177.9589) (59.9373, -178.1449) (60.0989, -178.3304) (60.2612, -178.5156) (60.4242, -178.7003) (60.5879, -178.8846) (60.7524, -179.0684) (60.9506, -179.2886) (61.1167, -179.4715) (61.2501, -179.6175) (61.3505, -179.7268) (61.4176, -179.7995) knots 0.383497 0.383497 0.383497 0.383497 0.383497 0.383497 0.385714 0.4 0.414286 0.428571 0.442857 0.457143 0.471429 0.485714 0.5 0.514286 0.528571 0.542857 0.557143 0.571429 0.585714 0.6 0.614286 0.628571 0.642857 0.657143 0.671429 0.685714 0.7 0.714286 0.728571 0.742857 0.757143 0.771429 0.785714 0.8 0.814286 0.828571 0.842857 0.857143 0.871429 0.885714 0.9 0.914286 0.928571 0.942857 0.957143 0.971429 1 1 1 1 1 1
  arc A5 (61.4176, -179.7995) -> (65.1686, -178.4742) centre (0, 0) ccw
  spline S10 degree 5 poles (65.0324, -167.9648) (65.0332, -167.9722) (65.039, -168.0274) (65.0496, -168.1304) (65.0648, -168.2813) (65.084, -168.4802) (65.106, -168.7198) (65.1268, -168.9598) (65.1466, -169.1999) (65.1652, -169.4404) (65.1827, -169.681) (65.1991, -169.922) (65.2145, -170.1631) (65.2288, -170.4046) (65.242, -170.6462) (65.2542, -170.8881) (65.2654, -171.1302) (65.2756, -171.3725) (65.2848, -171.615) (65.293, -171.8577) (65.3002, -172.1006) (65.3065, -172.3437) (65.3118, -172.587) (65.3161, -172.8305) (65.3195, -173.0742) (65.3219, -173.318) (65.3234, -173.5621) (65.324, -173.8063) (65.3237, -174.0506) (65.3225, -174.2952) (65.3204, -174.5398) (65.3173, -174.7847) (65.3134, -175.0297) (65.3086, -175.2749) (65.303, -175.5202) (65.2964, -175.7656) (65.289, -176.0112) (65.2808, -176.2569) (65.2717, -176.5028) (65.2617, -176.7488) (65.2509, -176.9949) (65.2393, -177.2411) (65.2268, -177.4875) (65.2109, -177.7833) (65.1966, -178.03) (65.1845, -178.2274) (65.175, -178.3755) (65.1686, -178.4742) knots 0.383497 0.383497 0.383497 0.383497 0.383497 0.383497 0.385714 0.4 0.414286 0.428571 0.442857 0.457143 0.471429 0.485714 0.5 0.514286 0.528571 0.542857 0.557143 0.571429 0.585714 0.6 0.614286 0.628571 0.642857 0.657143 0.671429 0.685714 0.7 0.714286 0.728571 0.742857 0.757143 0.771429 0.785714 0.8 0.814286 0.828571 0.842857 0.857143 0.871429 0.885714 0.9 0.914286 0.928571 0.942857 0.957143 0.971429 1 1 1 1 1 1
  spline S11 degree 3 poles (66.0255, -166.3233) (65.6608, -166.4681) (65.1243, -166.9682) (65.0016, -167.6721) (65.0324, -167.9648) knots 0 0 0 0 0.571429 1 1 1 1
  arc A6 (66.0255, -166.3233) -> (67.4181, -165.7637) centre (0, 0) ccw
  spline S12 degree 3 poles (69.2708, -166.2616) (69.0905, -166.0291) (68.5149, -165.6058) (67.7816, -165.6159) (67.4181, -165.7637) knots 0 0 0 0 0.428571 1 1 1 1
  spline S13 degree 5 poles (69.2708, -166.2616) (69.2754, -166.2675) (69.3094, -166.3114) (69.373, -166.3931) (69.4664, -166.5126) (69.5902, -166.6695) (69.7401, -166.8577) (69.8911, -167.0453) (70.0431, -167.2323) (70.196, -167.4188) (70.3499, -167.6047) (70.5047, -167.79) (70.6605, -167.9747) (70.8172, -168.1589) (70.9749, -168.3426) (71.1334, -168.5256) (71.2928, -168.7082) (71.4531, -168.8901) (71.6143, -169.0716) (71.7763, -169.2525) (71.9392, -169.4328) (72.1029, -169.6127) (72.2674, -169.792) (72.4328, -169.9708) (72.599, -170.149) (72.7659, -170.3268) (72.9337, -170.504) (73.1022, -170.6807) (73.2715, -170.8569) (73.4416, -171.0326) (73.6125, -171.2078) (73.7841, -171.3825) (73.9564, -171.5567) (74.1295, -171.7303) (74.3033, -171.9035) (74.4779, -172.0762) (74.6532, -172.2484) (74.8292, -172.4201) (75.0059, -172.5913) (75.1833, -172.762) (75.3613, -172.9322) (75.5401, -173.1019) (75.7196, -173.2712) (75.9358, -173.4737) (76.1168, -173.6419) (76.2621, -173.776) (76.3714, -173.8764) (76.4444, -173.9432) knots 0.383497 0.383497 0.383497 0.383497 0.383497 0.383497 0.385714 0.4 0.414286 0.428571 0.442857 0.457143 0.471429 0.485714 0.5 0.514286 0.528571 0.542857 0.557143 0.571429 0.585714 0.6 0.614286 0.628571 0.642857 0.657143 0.671429 0.685714 0.7 0.714286 0.728571 0.742857 0.757143 0.771429 0.785714 0.8 0.814286 0.828571 0.842857 0.857143 0.871429 0.885714 0.9 0.914286 0.928571 0.942857 0.957143 0.971429 1 1 1 1 1 1
  arc A7 (76.4444, -173.9432) -> (80.0695, -172.3046) centre (0, 0) ccw
  spline S14 degree 5 poles (79.0425, -161.8446) (79.0439, -161.8519) (79.0544, -161.9064) (79.0737, -162.0081) (79.1016, -162.1572) (79.1377, -162.3537) (79.1799, -162.5907) (79.221, -162.8279) (79.261, -163.0656) (79.2999, -163.3036) (79.3378, -163.5419) (79.3746, -163.7806) (79.4104, -164.0196) (79.4451, -164.2589) (79.4788, -164.4985) (79.5115, -164.7385) (79.5432, -164.9788) (79.5739, -165.2193) (79.6036, -165.4602) (79.6323, -165.7013) (79.6601, -165.9428) (79.687, -166.1845) (79.7129, -166.4264) (79.7378, -166.6687) (79.7619, -166.9112) (79.785, -167.154) (79.8072, -167.397) (79.8285, -167.6402) (79.8489, -167.8838) (79.8684, -168.1275) (79.8871, -168.3715) (79.9048, -168.6157) (79.9217, -168.8602) (79.9377, -169.1049) (79.9529, -169.3498) (79.9672, -169.5949) (79.9806, -169.8402) (79.9932, -170.0858) (80.005, -170.3315) (80.016, -170.5775) (80.0261, -170.8236) (80.0354, -171.07) (80.0439, -171.3165) (80.0531, -171.6126) (80.0597, -171.8595) (80.0644, -172.0573) (80.0675, -172.2057) (80.0695, -172.3046) knots 0.383497 0.383497 0.383497 0.383497 0.383497 0.383497 0.385714 0.4 0.414286 0.428571 0.442857 0.457143 0.471429 0.485714 0.5 0.514286 0.528571 0.542857 0.557143 0.571429 0.585714 0.6 0.614286 0.628571 0.642857 0.657143 0.671429 0.685714 0.7 0.714286 0.728571 0.742857 0.757143 0.771429 0.785714 0.8 0.814286 0.828571 0.842857 0.857143 0.871429 0.885714 0.9 0.914286 0.928571 0.942857 0.957143 0.971429 1 1 1 1 1 1
  spline S15 degree 3 poles (79.8928, -160.1248) (79.5417, -160.3) (79.0496, -160.8438) (78.987, -161.5556) (79.0425, -161.8446) knots 0 0 0 0 0.571429 1 1 1 1
  arc A8 (79.8928, -160.1248) -> (81.233, -159.4491) centre (0, 0) ccw
  spline S16 degree 3 poles (83.1213, -159.7881) (82.9219, -159.5716) (82.3124, -159.1987) (81.5826, -159.271) (81.233, -159.4491) knots 0 0 0 0 0.428571 1 1 1 1
  spline S17 degree 5 poles (83.1213, -159.7881) (83.1263, -159.7936) (83.1639, -159.8344) (83.2342, -159.9104) (83.3374, -160.0215) (83.4741, -160.1674) (83.6394, -160.3422) (83.8058, -160.5163) (83.973, -160.6898) (84.1412, -160.8626) (84.3103, -161.0348) (84.4803, -161.2063) (84.6512, -161.3772) (84.823, -161.5474) (84.9956, -161.717) (85.1691, -161.886) (85.3434, -162.0543) (85.5186, -162.2221) (85.6946, -162.3892) (85.8714, -162.5557) (86.0489, -162.7216) (86.2273, -162.8869) (86.4065, -163.0516) (86.5864, -163.2157) (86.7671, -163.3793) (86.9485, -163.5422) (87.1307, -163.7046) (87.3136, -163.8663) (87.4973, -164.0275) (87.6816, -164.1882) (87.8667, -164.3482) (88.0525, -164.5077) (88.239, -164.6667) (88.4262, -164.825) (88.6141, -164.9829) (88.8027, -165.1401) (88.9919, -165.2968) (89.1818, -165.453) (89.3724, -165.6086) (89.5636, -165.7636) (89.7555, -165.9181) (89.9481, -166.0721) (90.1412, -166.2255) (90.3738, -166.409) (90.5684, -166.5612) (90.7246, -166.6825) (90.842, -166.7733) (90.9204, -166.8337) knots 0.383497 0.383497 0.383497 0.383497 0.383497 0.383497 0.385714 0.4 0.414286 0.428571 0.442857 0.457143 0.471429 0.485714 0.5 0.514286 0.528571 0.542857 0.557143 0.571429 0.585714 0.6 0.614286 0.628571 0.642857 0.657143 0.671429 0.685714 0.7 0.714286 0.728571 0.742857 0.757143 0.771429 0.785714 0.8 0.814286 0.828571 0.842857 0.857143 0.871429 0.885714 0.9 0.914286 0.928571 0.942857 0.957143 0.971429 1 1 1 1 1 1
  arc A9 (90.9204, -166.8337) -> (94.3935, -164.8935) centre (0, 0) ccw
  spline S18 degree 5 poles (92.4831, -154.5582) (92.4852, -154.5654) (92.5002, -154.6188) (92.5281, -154.7186) (92.5686, -154.8647) (92.6211, -155.0575) (92.6833, -155.29) (92.7444, -155.5229) (92.8044, -155.7563) (92.8634, -155.9901) (92.9213, -156.2244) (92.9782, -156.4591) (93.0341, -156.6942) (93.089, -156.9297) (93.1429, -157.1657) (93.1958, -157.402) (93.2478, -157.6387) (93.2988, -157.8758) (93.3488, -158.1133) (93.3979, -158.3511) (93.4461, -158.5893) (93.4933, -158.8279) (93.5397, -159.0668) (93.5851, -159.306) (93.6296, -159.5456) (93.6732, -159.7855) (93.716, -160.0258) (93.7578, -160.2664) (93.7988, -160.5073) (93.8389, -160.7485) (93.8782, -160.9901) (93.9166, -161.2319) (93.9541, -161.474) (93.9908, -161.7165) (94.0267, -161.9592) (94.0617, -162.2022) (94.096, -162.4455) (94.1293, -162.6891) (94.1619, -162.933) (94.1937, -163.1771) (94.2246, -163.4215) (94.2548, -163.6662) (94.2842, -163.9111) (94.3184, -164.2054) (94.346, -164.4509) (94.3674, -164.6475) (94.3832, -164.7951) (94.3935, -164.8935) knots 0.383497 0.383497 0.383497 0.383497 0.383497 0.383497 0.385714 0.4 0.414286 0.428571 0.442857 0.457143 0.471429 0.485714 0.5 0.514286 0.528571 0.542857 0.557143 0.571429 0.585714 0.6 0.614286 0.628571 0.642857 0.657143 0.671429 0.685714 0.7 0.714286 0.728571 0.742857 0.757143 0.771429 0.785714 0.8 0.814286 0.828571 0.842857 0.857143 0.871429 0.885714 0.9 0.914286 0.928571 0.942857 0.957143 0.971429 1 1 1 1 1 1
  spline S19 degree 3 poles (93.1845, -152.7726) (92.8495, -152.9769) (92.4054, -153.5605) (92.4034, -154.275) (92.4831, -154.5582) knots 0 0 0 0 0.571429 1 1 1 1
  arc A10 (93.1845, -152.7726) -> (94.4626, -151.9857) centre (0, 0) ccw
  spline S20 degree 3 poles (96.3728, -152.1633) (96.1558, -151.9645) (95.5169, -151.6446) (94.7958, -151.7785) (94.4626, -151.9857) knots 0 0 0 0 0.428571 1 1 1 1
  spline S21 degree 5 poles (96.3728, -152.1633) (96.3783, -152.1683) (96.4192, -152.2058) (96.4957, -152.2756) (96.608, -152.3776) (96.7565, -152.5113) (96.9361, -152.6715) (97.1166, -152.8309) (97.298, -152.9895) (97.4802, -153.1475) (97.6633, -153.3047) (97.8472, -153.4611) (98.032, -153.6169) (98.2176, -153.7719) (98.404, -153.9263) (98.5912, -154.0799) (98.7792, -154.2329) (98.9679, -154.3852) (99.1574, -154.5368) (99.3477, -154.6877) (99.5387, -154.8379) (99.7304, -154.9875) (99.9229, -155.1364) (100.1161, -155.2847) (100.31, -155.4323) (100.5046, -155.5793) (100.6999, -155.7256) (100.8959, -155.8713) (101.0926, -156.0164) (101.2899, -156.1608) (101.4879, -156.3046) (101.6865, -156.4477) (101.8858, -156.5903) (102.0858, -156.7322) (102.2864, -156.8735) (102.4876, -157.0142) (102.6895, -157.1543) (102.8919, -157.2938) (103.095, -157.4326) (103.2987, -157.5709) (103.503, -157.7086) (103.7079, -157.8457) (103.9134, -157.9822) (104.1607, -158.1452) (104.3675, -158.2804) (104.5334, -158.388) (104.6581, -158.4685) (104.7414, -158.5221) knots 0.383497 0.383497 0.383497 0.383497 0.383497 0.383497 0.385714 0.4 0.414286 0.428571 0.442857 0.457143 0.471429 0.485714 0.5 0.514286 0.528571 0.542857 0.557143 0.571429 0.585714 0.6 0.614286 0.628571 0.642857 0.657143 0.671429 0.685714 0.7 0.714286 0.728571 0.742857 0.757143 0.771429 0.785714 0.8 0.814286 0.828571 0.842857 0.857143 0.871429 0.885714 0.9 0.914286 0.928571 0.942857 0.957143 0.971429 1 1 1 1 1 1
  arc A11 (104.7414, -158.5221) -> (108.0374, -156.2944) centre (0, 0) ccw
  spline S22 degree 5 poles (105.2574, -146.1583) (105.26, -146.1653) (105.2796, -146.2173) (105.3158, -146.3143) (105.3685, -146.4565) (105.4373, -146.6441) (105.5189, -146.8705) (105.5995, -147.0974) (105.6791, -147.3248) (105.7577, -147.5528) (105.8353, -147.7813) (105.9119, -148.0103) (105.9876, -148.2399) (106.0622, -148.4699) (106.1359, -148.7004) (106.2087, -148.9314) (106.2806, -149.1628) (106.3515, -149.3947) (106.4215, -149.6271) (106.4906, -149.8599) (106.5588, -150.0932) (106.6261, -150.3269) (106.6925, -150.561) (106.758, -150.7955) (106.8227, -151.0305) (106.8865, -151.2659) (106.9495, -151.5016) (107.0116, -151.7378) (107.0728, -151.9744) (107.1333, -152.2113) (107.1929, -152.4487) (107.2516, -152.6864) (107.3096, -152.9245) (107.3667, -153.1629) (107.4231, -153.4017) (107.4786, -153.6409) (107.5333, -153.8804) (107.5872, -154.1203) (107.6404, -154.3605) (107.6927, -154.6011) (107.7443, -154.842) (107.7951, -155.0832) (107.8451, -155.3248) (107.9042, -155.6151) (107.9525, -155.8573) (107.9906, -156.0514) (108.0187, -156.1971) (108.0374, -156.2944) knots 0.383497 0.383497 0.383497 0.383497 0.383497 0.383497 0.385714 0.4 0.414286 0.428571 0.442857 0.457143 0.471429 0.485714 0.5 0.514286 0.528571 0.542857 0.557143 0.571429 0.585714 0.6 0.614286 0.628571 0.642857 0.657143 0.671429 0.685714 0.7 0.714286 0.728571 0.742857 0.757143 0.771429 0.785714 0.8 0.814286 0.828571 0.842857 0.857143 0.871429 0.885714 0.9 0.914286 0.928571 0.942857 0.957143 0.971429 1 1 1 1 1 1
  spline S23 degree 3 poles (105.8048, -144.3196) (105.4884, -144.5516) (105.0953, -145.1707) (105.1539, -145.8829) (105.2574, -146.1583) knots 0 0 0 0 0.571429 1 1 1 1
  arc A12 (105.8048, -144.3196) -> (107.0115, -143.4271) centre (0, 0) ccw
  spline S24 degree 3 poles (108.93, -143.4421) (108.6969, -143.2625) (108.0331, -142.9979) (107.326, -143.1925) (107.0115, -143.4271) knots 0 0 0 0 0.428571 1 1 1 1
  spline S25 degree 5 poles (108.93, -143.4421) (108.9359, -143.4467) (108.9798, -143.4806) (109.062, -143.5436) (109.1825, -143.6357) (109.3418, -143.7563) (109.5343, -143.9007) (109.7277, -144.0442) (109.9219, -144.1869) (110.1168, -144.3288) (110.3126, -144.47) (110.5091, -144.6103) (110.7065, -144.7498) (110.9045, -144.8885) (111.1033, -145.0265) (111.3029, -145.1637) (111.5032, -145.3002) (111.7042, -145.4359) (111.9058, -145.5709) (112.1082, -145.7051) (112.3113, -145.8386) (112.515, -145.9714) (112.7194, -146.1035) (112.9245, -146.2348) (113.1302, -146.3655) (113.3366, -146.4954) (113.5436, -146.6247) (113.7512, -146.7532) (113.9595, -146.8811) (114.1683, -147.0082) (114.3778, -147.1347) (114.5879, -147.2605) (114.7986, -147.3856) (115.0098, -147.5101) (115.2217, -147.6339) (115.4341, -147.757) (115.6471, -147.8795) (115.8607, -148.0013) (116.0748, -148.1224) (116.2895, -148.2429) (116.5048, -148.3628) (116.7206, -148.482) (116.9369, -148.6006) (117.1971, -148.7421) (117.4146, -148.8592) (117.5891, -148.9524) (117.7202, -149.022) (117.8077, -149.0683) knots 0.383497 0.383497 0.383497 0.383497 0.383497 0.383497 0.385714 0.4 0.414286 0.428571 0.442857 0.457143 0.471429 0.485714 0.5 0.514286 0.528571 0.542857 0.557143 0.571429 0.585714 0.6 0.614286 0.628571 0.642857 0.657143 0.671429 0.685714 0.7 0.714286 0.728571 0.742857 0.757143 0.771429 0.785714 0.8 0.814286 0.828571 0.842857 0.857143 0.871429 0.885714 0.9 0.914286 0.928571 0.942857 0.957143 0.971429 1 1 1 1 1 1
  arc A13 (117.8077, -149.0683) -> (120.9029, -146.5691) centre (0, 0) ccw
  spline S26 degree 5 poles (117.2733, -136.7053) (117.2765, -136.7121) (117.3004, -136.7622) (117.3447, -136.8558) (117.4093, -136.993) (117.4937, -137.1741) (117.5943, -137.3927) (117.6938, -137.612) (117.7924, -137.8319) (117.8901, -138.0524) (117.9868, -138.2735) (118.0825, -138.4952) (118.1774, -138.7175) (118.2713, -138.9403) (118.3643, -139.1637) (118.4564, -139.3877) (118.5476, -139.6122) (118.6379, -139.8373) (118.7274, -140.0629) (118.8159, -140.289) (118.9037, -140.5157) (118.9906, -140.7428) (119.0766, -140.9705) (119.1618, -141.1986) (119.2462, -141.4272) (119.3297, -141.6563) (119.4124, -141.8859) (119.4943, -142.116) (119.5754, -142.3465) (119.6558, -142.5774) (119.7353, -142.8089) (119.814, -143.0407) (119.8919, -143.2731) (119.9691, -143.5058) (120.0454, -143.739) (120.1211, -143.9726) (120.1959, -144.2066) (120.27, -144.441) (120.3433, -144.6759) (120.4159, -144.9112) (120.4877, -145.1468) (120.5587, -145.3829) (120.6291, -145.6193) (120.7126, -145.9035) (120.7813, -146.1409) (120.8356, -146.331) (120.876, -146.4738) (120.9029, -146.5691) knots 0.383497 0.383497 0.383497 0.383497 0.383497 0.383497 0.385714 0.4 0.414286 0.428571 0.442857 0.457143 0.471429 0.485714 0.5 0.514286 0.528571 0.542857 0.557143 0.571429 0.585714 0.6 0.614286 0.628571 0.642857 0.657143 0.671429 0.685714 0.7 0.714286 0.728571 0.742857 0.757143 0.771429 0.785714 0.8 0.814286 0.828571 0.842857 0.857143 0.871429 0.885714 0.9 0.914286 0.928571 0.942857 0.957143 0.971429 1 1 1 1 1 1
  spline S27 degree 3 poles (117.6628, -134.8268) (117.3672, -135.0848) (117.028, -135.7351) (117.1468, -136.4396) (117.2733, -136.7053) knots 0 0 0 0 0.571429 1 1 1 1
  arc A14 (117.6628, -134.8268) -> (118.7895, -133.8352) centre (0, 0) ccw
  spline S28 degree 3 poles (120.7023, -133.6875) (120.4548, -133.5282) (119.771, -133.3209) (119.083, -133.5748) (118.7895, -133.8352) knots 0 0 0 0 0.428571 1 1 1 1
  spline S29 degree 5 poles (120.7023, -133.6875) (120.7086, -133.6915) (120.7552, -133.7215) (120.8424, -133.7774) (120.9703, -133.8589) (121.1393, -133.9656) (121.3433, -134.0931) (121.5482, -134.2197) (121.7538, -134.3455) (121.9601, -134.4703) (122.1671, -134.5943) (122.3748, -134.7175) (122.5833, -134.8398) (122.7924, -134.9612) (123.0022, -135.0818) (123.2127, -135.2016) (123.4238, -135.3206) (123.6356, -135.4388) (123.848, -135.5562) (124.061, -135.6728) (124.2747, -135.7886) (124.4889, -135.9036) (124.7038, -136.0179) (124.9193, -136.1314) (125.1353, -136.2441) (125.352, -136.3561) (125.5692, -136.4673) (125.787, -136.5777) (126.0053, -136.6875) (126.2242, -136.7965) (126.4437, -136.9047) (126.6637, -137.0123) (126.8842, -137.1191) (127.1053, -137.2252) (127.3268, -137.3305) (127.5489, -137.4352) (127.7716, -137.5392) (127.9947, -137.6424) (128.2183, -137.745) (128.4425, -137.8468) (128.6671, -137.948) (128.8922, -138.0485) (129.1178, -138.1483) (129.3891, -138.2672) (129.6158, -138.3655) (129.7975, -138.4435) (129.934, -138.5018) (130.0251, -138.5405) knots 0.383497 0.383497 0.383497 0.383497 0.383497 0.383497 0.385714 0.4 0.414286 0.428571 0.442857 0.457143 0.471429 0.485714 0.5 0.514286 0.528571 0.542857 0.557143 0.571429 0.585714 0.6 0.614286 0.628571 0.642857 0.657143 0.671429 0.685714 0.7 0.714286 0.728571 0.742857 0.757143 0.771429 0.785714 0.8 0.814286 0.828571 0.842857 0.857143 0.871429 0.885714 0.9 0.914286 0.928571 0.942857 0.957143 0.971429 1 1 1 1 1 1
  arc A15 (130.0251, -138.5405) -> (132.8972, -135.7878) centre (0, 0) ccw
  spline S30 degree 5 poles (128.4443, -126.2674) (128.448, -126.2738) (128.476, -126.3217) (128.5282, -126.4112) (128.6042, -126.5424) (128.7036, -126.7158) (128.8224, -126.9251) (128.9402, -127.1351) (129.0571, -127.3458) (129.173, -127.5573) (129.2881, -127.7694) (129.4024, -127.9821) (129.5157, -128.1956) (129.6282, -128.4097) (129.7398, -128.6244) (129.8505, -128.8398) (129.9605, -129.0558) (130.0695, -129.2724) (130.1778, -129.4895) (130.2852, -129.7073) (130.3919, -129.9257) (130.4977, -130.1447) (130.6027, -130.3642) (130.707, -130.5843) (130.8104, -130.8049) (130.9131, -131.0261) (131.015, -131.2479) (131.1161, -131.4702) (131.2165, -131.693) (131.3161, -131.9163) (131.415, -132.1401) (131.5131, -132.3645) (131.6104, -132.5894) (131.707, -132.8147) (131.8029, -133.0406) (131.898, -133.2669) (131.9925, -133.4938) (132.0862, -133.7211) (132.1791, -133.9489) (132.2714, -134.1771) (132.3629, -134.4059) (132.4538, -134.635) (132.5439, -134.8647) (132.6512, -135.1408) (132.7398, -135.3714) (132.81, -135.5563) (132.8624, -135.6951) (132.8972, -135.7878) knots 0.383497 0.383497 0.383497 0.383497 0.383497 0.383497 0.385714 0.4 0.414286 0.428571 0.442857 0.457143 0.471429 0.485714 0.5 0.514286 0.528571 0.542857 0.557143 0.571429 0.585714 0.6 0.614286 0.628571 0.642857 0.657143 0.671429 0.685714 0.7 0.714286 0.728571 0.742857 0.757143 0.771429 0.785714 0.8 0.814286 0.828571 0.842857 0.857143 0.871429 0.885714 0.9 0.914286 0.928571 0.942857 0.957143 0.971429 1 1 1 1 1 1